# Autodesk Inventor part: m2_bolt_5mm
Saved by Autodesk Inventor 2021 (Build 250183000, 183)
## iProperties
Created: 2021-03-15
Part Number: m2_bolt_5mm
Material: Stainless Steel
Document SubType Name: Modeling
Designer: Tomasz Lisowski
Density: 8 g/cm^3
Appearance: Semi-Polished
Author: Tomasz Lisowski
Autodesk Inventor part; units mm, degrees
ref_plane "YZ Plane" through (0, 0, 0) normal (1, 0, 0) x (0, 1, 0)
ref_plane "XZ Plane" through (0, 0, 0) normal (0, 1, 0) x (-1, 0, 0)
ref_plane "XY Plane" through (0, 0, 0) normal (0, 0, 1) x (1, 0, 0)
sketch "Sketch1" plane through (0, 0, 0) normal (0, 1, 0) x (-1, 0, 0)
  circle A0 centre (0, 0) radius 2.25
  dimension "d0" = 4.5
  constraints: 1 centre point, 1 coincident
  measures "d0" diameter of A0
extrude "Extrusion1" add sketch "Sketch1" along normal blind 2.5
sketch "Sketch2" plane through (0, 2.5, 0) normal (0, 1, 0) x (1, 0, 0)
  circle A0 centre (0, 0) radius 1
  dimension "d3" = 2
  constraints: 1 centre point, 1 coincident
  measures "d3" diameter of A0
extrude "Extrusion2" add sketch "Sketch2" along normal blind 5
sketch "Sketch3" plane through (0, 0, 0) normal (0, -1, 0) x (1, 0, 0)
  line L0 (0, -1.1547) -> (-1, -0.5774)
  line L1 (-1, -0.5774) -> (-1, 0.5774)
  line L2 (-1, 0.5774) -> (0, 1.1547)
  line L3 (0, 1.1547) -> (1, 0.5774)
  line L4 (1, 0.5774) -> (1, -0.5774)
  line L5 (1, -0.5774) -> (0, -1.1547)
  point P0 (0, 0)
  point P1 (0, 0)
  dimension "d6" = 2
  constraints: 12 end point, 1 coincident, 1 vertical alignment, 13 other
  measures "d6" distance between parallel lines of L1 L4
extrude "Extrusion3" cut sketch "Sketch3" against normal blind 1
body "Solid1"
